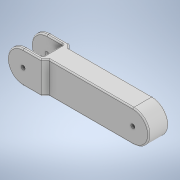
# Autodesk Inventor part: Arm1
Saved by Autodesk Inventor 2021 (Build 250183000, 183)
## iProperties
Created: 2024-09-30
Part Number: Arm1
Material: Generic
Document SubType Name: Modeling
Designer: Swoby
Density: 1 g/cm^3
Appearance: Default
Author: Swoby
Autodesk Inventor part; units mm, degrees
ref_plane "YZ Plane" through (0, 0, 0) normal (1, 0, 0) x (0, 1, 0)
ref_plane "XZ Plane" through (0, 0, 0) normal (0, 1, 0) x (-1, 0, 0)
ref_plane "XY Plane" through (0, 0, 0) normal (0, 0, 1) x (1, 0, 0)
sketch "Sketch1" plane through (0, 0, 0) normal (0, 0, 1) x (1, 0, 0)
  arc A0 (0, 40) -> (0, -40) centre (0, 0) ccw
  arc A1 (265, -40) -> (265, 40) centre (265, 0) ccw
  line L0 (0, 0) -> (265, 0) construction
  line L1 (0, 40) -> (265, 40)
  line L2 (0, -40) -> (265, -40)
  arc A2 (40, 0) -> (0, 40) centre (0, 0) ccw construction
  arc A3 (0, -40) -> (40, 0) centre (0, 0) ccw construction
  arc A4 (225, 0) -> (265, -40) centre (265, 0) ccw construction
  arc A5 (265, 40) -> (225, 0) centre (265, 0) ccw construction
  circle A6 centre (0, 0) radius 5
  circle A7 centre (265, 0) radius 5
  dimension "d0" = 80
  dimension "d1" = 80
  dimension "d2" = 265
  dimension "d3" = 10
  dimension "d4" = 10
  constraints: 12 point on circle, 8 centre point, 8 tangent, 6 end point, 4 coincident, 2 point on line, 1 horizontal
  measures "d0" diameter of A0
  measures "d1" diameter of A1
  measures "d2" distance of L0.start L0.end
  measures "d3" diameter of A6
  measures "d4" diameter of A7
extrude "Extrusion1" add sketch "Sketch1" along normal mid plane 70
sketch "Sketch2" plane through (0, 40, 35) normal (0, 1, 0) x (1, 0, 0)
  line L0 (-40, 0) -> (0, 0) construction
  line L1 (-40, 0) -> (45, 0) construction
  line L2 (45, 70) -> (45, 69.4311) construction
  line L3 (305, 70) -> (305, 0) construction
  line L4 (55, 10) -> (305, 10) construction
  line L5 (305, 10) -> (305, 60) construction
  line L6 (305, 60) -> (55, 60) construction
  line L7 (45, 60) -> (45, 10) construction
  line L8 (0, 70) -> (265, 70) construction
  line L9 (265, 0) -> (0, 0) construction
  line L10 (45, 60) -> (305, 60) construction
  line L11 (305, 60) -> (305, 70)
  line L12 (305, 70) -> (45, 70)
  line L13 (45, 70) -> (45, 60) construction
  line L14 (45, 10) -> (305, 10) construction
  line L15 (305, 10) -> (305, 0)
  line L16 (305, 0) -> (45, 0)
  line L17 (45, 0) -> (45, 0)
  line L18 (55, 60) -> (45, 70)
  line L19 (55, 10) -> (45, 0)
  line L20 (55, 60) -> (305, 60)
  line L21 (305, 10) -> (50, 10)
  line L22 (-40, 70) -> (-40, 0) projected
  line L23 (-40, 10) -> (40, 10)
  line L24 (40, 10) -> (40, 60)
  line L25 (40, 60) -> (-40, 60)
  line L26 (-40, 60) -> (-40, 10)
  point P0 (0, 35)
  point P1 (45, 70)
  point P2 (45, 0)
  point P3 (55, 10)
  dimension "d7" = 85
  dimension "d8" = 10
  dimension "d9" = 10
  dimension "d10" = 10
  dimension "d11" = 10
  dimension "d12" = 10
  dimension "d13" = 10
  dimension "d14" = 80
  constraints: 44 end point, 12 point on line, 8 parallel, 5 perpendicular, 4 collinear, 4 horizontal
  measures "d7" distance of L0.start L1.end
  measures "d8" distance between parallel lines of L6 L8
  measures "d9" distance between parallel lines of L9 L4
  measures "d10" distance of L6.end point (45, 60)
  measures "d11" distance of L2.start point (45, 60)
  measures "d12" distance of L4.start L7.end
  measures "d13" distance of L17.end L7.end
  measures "d14" distance between parallel lines of L26 L24
extrude "Extrusion2" cut sketch "Sketch2" against normal through all
fillet "Fillet1" radius 3 26 edges at (305, 0, 25) (160, -40, 25) (160, 40, 25) (305, 0, -25) (160, -40, -25) (160, 40, -25) (-40, 0, 35) (22.5, -40, 35) (22.5, 40, 35) (-40, 0, 25) (20, -40, 25) (20, 40, 25) (-40, 0, -25) (20, -40, -25) (20, 40, -25) (-40, 0, -35) (22.5, -40, -35) (22.5, 40, -35) (40, 40, 0) (40, -40, 0) (50, -40, 30) (50, 40, 30) (50, 40, -30) (50, -40, -30) (40, 0, -25) (40, 0, 25)
equation "\"d11\" = d10"
equation "\"d12\" = d10"
equation "\"d13\" = d12"
body "Solid1"
